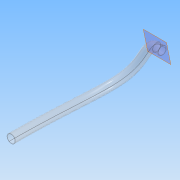
# Autodesk Inventor part: Top_LHS Pipe
Saved by Autodesk Inventor 2018.1 (Build 221171000, 171)
## iProperties
Created: 2019-03-19
Part Number: Top_LHS Pipe
Material: PMMA Plastic
Document SubType Name: Modeling
Designer: James
Density: 1.188 g/cm^3
Appearance: Polycarbonate - Clear
Author: James
Autodesk Inventor part; units mm, degrees
ref_plane "YZ Plane" through (0, 0, 0) normal (1, 0, 0) x (0, 1, 0)
ref_plane "XY Plane" through (0, 0, 0) normal (0, 0, 1) x (1, 0, 0)
sketch "Sketch2" plane through (0, 0, 0) normal (1, 0, 0) x (0, 1, 0)
  circle A0 centre (0, 0) radius 20
  circle A1 centre (0, 0) radius 23
  dimension "d2" = 40
  dimension "d3" = 46
  constraints: 2 centre point, 2 coincident
  measures "d2" diameter of A0
  measures "d3" diameter of A1
sketch3d "3D Sketch1"
  spline S0 degree 4 poles (0, 0, 0) (-80, 0, 0) (-80, 0, -215) (-180, 0, -215) (-180, -600, -215) knots 1 1 1 1 1 2 2 2 2 2
  dimension "d4" = 80
  dimension "d5" = 215
  dimension "d6" = 100
  dimension "d7" = 600
sweep "Sweep1" add profiles "Sketch2" path "3D Sketch1"
sketch "Sketch3" plane through (0, 0, 0) normal (1, 0, 0) x (0, 0, -1)
  spline S0 degree 6 poles (0, 20) (33.2309, 20) (38.0022, -21.091) (0, -54.9823) (-38.0022, -21.091) (-33.2309, 20) (0, 20) knots 0 0 0 0 0 0 0 1 1 1 1 1 1 1 weights 1.669078 1.03673 1.038347 0.853534 1.038347 1.03673 1.669078 projected
  circle A0 centre (0, 0) radius 23 projected
  point P0 (0, 23)
  constraints: 1 vertical alignment, 1 other
extrude "Extrusion1" add sketch "Sketch3" along normal blind 30
ref_plane "Work Plane1" through (0, 0, 0) normal (0, 0.9799247, 0.1993679) x (1, 0, 0)
sketch "Sketch4" plane through (0, 0, 0) normal (0, 0.9799247, 0.1993679) x (1, 0, 0)
  line L0 (30, -23) -> (30, 23) projected
  line L1 (0, 23) -> (0, -23) projected
  point P0 (0, 0)
  point P1 (7.5, 0)
  point P2 (30, 0)
  point P3 (0, 4.5855)
  dimension "d23" = 7.5
  constraints: 1 horizontal alignment, 1 midpoint
  measures "d23" distance of point (7.5, 0) point (0, 0)
hole "Hole1" at (7.5, 0, 0) direction (0, 0.9799247, 0.1993679) diameter 4.5 end through all
body "Solid1"
